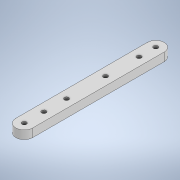
# Autodesk Inventor part: Base
Saved by Autodesk Inventor 2022 (Build 260153000, 153)
## iProperties
Created: 2022-02-12
Part Number: Base
Material: Generic
Document SubType Name: Modeling
Designer: juanp
Density: 1 g/cm^3
Appearance: Default
Author: juanp
Autodesk Inventor part; units mm, degrees
ref_plane "YZ Plane" through (0, 0, 0) normal (1, 0, 0) x (0, 1, 0)
ref_plane "XZ Plane" through (0, 0, 0) normal (0, 1, 0) x (-1, 0, 0)
ref_plane "XY Plane" through (0, 0, 0) normal (0, 0, 1) x (1, 0, 0)
sketch "Sketch1" plane through (0, 0, 0) normal (0, 1, 0) x (-1, 0, 0)
  line L0 (0, -78.504) -> (0, 78.504) construction
  line L1 (10, -78.504) -> (10, 78.504)
  line L2 (-10, 78.504) -> (-10, -78.504)
  arc A0 (-10, -78.504) -> (10, -78.504) centre (0, -78.504) ccw
  arc A1 (10, 78.504) -> (-10, 78.504) centre (0, 78.504) ccw
  circle A2 centre (0, 78.504) radius 10 construction
  circle A3 centre (0, -78.504) radius 10 construction
  circle A4 centre (0, -78.504) radius 2.65
  circle A5 centre (0, 78.504) radius 2.65
  circle A6 centre (0, 55.004) radius 2.65
  circle A7 centre (0, 28.004) radius 2.65
  circle A8 centre (0, -18.5134) radius 2.65
  circle A9 centre (0, -58.5134) radius 2.65
  point P0 (0, 0)
  point P1 (0, 68.504)
  point P2 (0, -68.504)
  dimension "d0" = 137.008
  dimension "d1" = 20
  dimension "d2" = 5.3
  dimension "d5" = 27
  dimension "d6" = 13.5
  dimension "d7" = 40
  dimension "d8" = 46.5174
  constraints: 8 centre point, 8 end point, 6 point on line, 5 equal radius, 4 coincident, 4 point on circle, 4 tangent, 2 vertical alignment, 1 midpoint, 1 parallel, 1 vertical, 6 other
  measures "d1" distance between parallel lines of L1 L2
  measures "d2" diameter of A4
  measures "d5" distance of A7.centre A6.centre
  measures "d6" distance of point (0, 68.504) A6.centre
  measures "d7" distance of A9.centre A8.centre
  measures "d8" distance of A8.centre A7.centre
extrude "Extrusion1" add sketch "Sketch1" along normal blind 10
body "Solid1"
